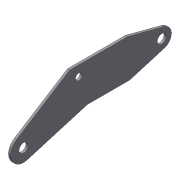
# Autodesk Inventor part: UPPER_LEG_OUTER_FRAME
Saved by Autodesk Inventor 2019.4 (Build 234330000, 330)
## iProperties
Created: 2019-11-12
Part Number: UPPER_LEG_OUTER_FRAME
Material: 一般
Document SubType Name: Modeling
Designer: y6tada
Density: 1 g/cm^3
Appearance: 既定
Author: y6tada
Autodesk Inventor part; units mm, degrees
ref_plane "YZ Plane" through (0, 0, 0) normal (1, 0, 0) x (0, 1, 0)
ref_plane "XZ Plane" through (0, 0, 0) normal (0, 1, 0) x (-1, 0, 0)
ref_plane "XY Plane" through (0, 0, 0) normal (0, 0, 1) x (1, 0, 0)
sketch "スケッチ1" plane through (0, 0, 0) normal (1, 0, 0) x (0, 1, 0)
  circle A0 centre (0, 0) radius 4
  line L0 (0, 0) -> (-22.5, 122.9583) construction
  circle A1 centre (-22.5, 122.9583) radius 4
  line L1 (8.2023, 76.9551) -> (-8.2023, 76.9551) construction
  line L2 (-8.2023, 76.9551) -> (-8.2023, 33.2653) construction
  line L3 (-8.2023, 33.2653) -> (8.2023, 33.2653) construction
  line L4 (8.2023, 33.2653) -> (8.2023, 76.9551) construction
  line L5 (0, 33.2653) -> (0, 0) construction
  line L6 (8.346, -2.1863) -> (16.9174, 30.5349)
  line L7 (16.9174, 30.5349) -> (16.9174, 81.9072)
  line L8 (16.9174, 81.9072) -> (-12.8803, 129.04)
  line L9 (-33.4087, 119.7141) -> (-17.491, 66.1909)
  line L10 (-17.491, 66.1909) -> (-17.491, 28.5475)
  line L11 (-17.491, 28.5475) -> (-8.2697, -2.4594)
  arc A2 (-12.8803, 129.04) -> (-33.4087, 119.7141) centre (-22.5, 122.9583) ccw
  arc A3 (-8.2697, -2.4594) -> (8.346, -2.1863) centre (0, 0) ccw
  circle A4 centre (7.6951, 73.7445) radius 3
  dimension "d0" = 8
  dimension "d1" = 8
  dimension "d2" = 125
  dimension "d3" = 22.5
  dimension "d6" = 6
  constraints: 24 end point, 5 centre point, 4 point on circle, 4 tangent, 3 parallel, 3 vertical, 2 coincident, 2 concentric, 1 horizontal, 1 midpoint, 1 perpendicular
  measures "d0" diameter of A0
  measures "d1" diameter of A1
  measures "d2" distance of L0.start L0.end
  measures "d3" horizontal distance of point (0, 0) L0.end
  measures "d6" diameter of A4
extrude "押し出し1" add sketch "スケッチ1" along normal blind 2
